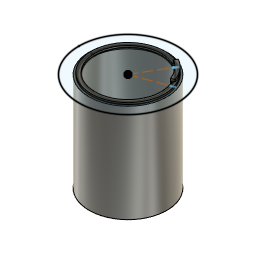
ex-vent v5 (Autodesk Fusion 360 design; units mm, degrees)
Autodesk Fusion 360 part; units mm, degrees
note: some values were not read from the file. Chosen so that the rebuilt part matches the saved one: the hand of a thread or coil.
sketch "Sketch1" plane through (0, 0, 0) normal (0, 0, 1) x (1, 0, 0)
  circle A0 centre (0, 0) radius 75.5
  circle A1 centre (0, 0) radius 79
  circle A2 centre (0, 0) radius 70
  line L0 (-75.5, 0) -> (75.5, 0)
  circle A3 centre (0, 0) radius 100
  dimension "ductid" = 151
  dimension "ductod" = 158
  dimension "d3" = 140
  dimension "d43" = 200
  constraint coincident A0.centre A1.centre
  constraint concentric A0 A2
  constraint coincident A0 L0.start
  constraint coincident A0 L0.end
  constraint horizontal L0
  constraint concentric A2 A3
  measures "ductid" diameter of A0
  measures "ductod" diameter of A1
  measures "d3" diameter of A2
  measures "d43" diameter of A3
extrude "Extrude1" add sketch "Sketch1" along normal blind 200 contours A1
sketch "Sketch2" plane through (0, 0, 200) normal (0, 0, 1) x (-1, 0, 0)
  circle A0 centre (0, 0) radius 75.5
  circle A1 centre (0, 0) radius 79
  circle A2 centre (0, 0) radius 75
  circle A3 centre (0, 0) radius 100
  circle A4 centre (0, 0) radius 72.5
  circle A5 centre (0, 0) radius 67.5
  circle A6 centre (0, 0) radius 69 construction
  arc A7 (-64.8289, -23.6266) -> (-34.4749, -59.7702) centre (0, 0) ccw
  line L0 (0, 0) -> (-64.8289, -23.6266) construction
  line L1 (0, 0) -> (-34.4749, -59.7702) construction
  line L2 (-64.8289, -23.6266) -> (-63.4196, -23.113)
  line L3 (-34.4749, -59.7702) -> (-33.7255, -58.4709)
  line L4 (-33.7255, -58.4709) -> (-36.2236, -62.8021)
  line L5 (-35.0164, -57.707) -> (-37.5152, -62.0392)
  line L6 (-36.2658, -59.8731) -> (-34.9745, -60.6365) construction
  line L7 (-63.4196, -23.113) -> (-68.1173, -24.8251)
  line L8 (-33.7255, -58.4709) -> (-37.5424, -64.9274)
  line L9 (-35.0164, -57.707) -> (-38.7645, -64.2052)
  line L10 (-63.4196, -23.113) -> (-70.4662, -25.6811)
  dimension "d13" = 200
  dimension "d14" = 145
  dimension "d17" = 150
  dimension "d20" = 135
  dimension "d21" = 138
  dimension "d22" = 40
  dimension "d23" = 1.5
  constraint coincident A0.centre A1.centre
  constraint concentric A2 A3
  constraint concentric A3 A5
  constraint coincident A6 A7.start
  constraint coincident A5 L2.end
  constraint coincident L0 L2.end
  constraint coincident L1 L3.end
  constraint coincident A5 L3.end
  constraint coincident A4 L4.end
  constraint parallel L3 L4
  constraint coincident A5 L5.start
  constraint coincident A4 L5.end
  constraint parallel L4 L5
  constraint midpoint L5 L6.start
  constraint midpoint L4 L6.end
  constraint coincident A4 L7.end
  constraint parallel L2 L7
  constraint coincident A2 L8.end
  constraint perpendicular L6 L8
  constraint coincident A2 L9.end
  constraint parallel L5 L9
  constraint coincident A2 L10.end
  constraint parallel L7 L10
  measures "d13" diameter of A3
  measures "d14" diameter of A4
  measures "d17" diameter of A2
  measures "d20" diameter of A5
  measures "d21" diameter of A6
  measures "d22" angle of L0 L1
  measures "d23" distance of L6.start L6.end
extrude "Extrude2" add sketch "Sketch2" against normal blind 5 contours A0 | A2 A4 L8 L10 | A2 A4 L9 L10 | A2 A4 L8 L9
extrude "Extrude3" add sketch "Sketch2" along normal blind 3.5 contours A2 A4 L8 L10 | A2 A4 L9 L10 | A2 A4 L8 L9 | A4 A7 L5 L7 L9 L10 | A4 A5 L2 L3 L4 L7 L10 | A4 A7 L4 L8 | A4 A7 L5 L8 L9 | A5 A7 L2 L5 L7 L9 L10 | A7 L3 L4 L8 | A5 A7 L5 L8 L9
extrude "Extrude4" add sketch "Sketch2" along normal blind 5.8 from surface at 3.5 contours A2 A4 L8 L9 | A4 A7 L5 L8 L9 | A5 A7 L2 L5 L7 L9 L10 | A5 A7 L5 L8 L9
extrude "Extrude5" add sketch "Sketch2" along normal blind 4.2 from surface at 9.3 contours A2 A4 L9 L10 | A2 A4 L8 L9 | A4 A7 L5 L7 L9 L10 | A4 A7 L5 L8 L9 | A5 A7 L2 L5 L7 L9 L10 | A5 A7 L5 L8 L9
chamfer "Chamfer3" distance 3 angle 45 1 edges at (-70.3907, -27.302, 195)
chamfer "Chamfer4" distance 5 angle 45 1 edges at (67.5937, -26.2171, 200)
coil "CoilPrimitive1" add diameter 150 section triangle in size 6 on centre turns 4 pitch 5 left hand placed x (1, 0, 0) y (0, 1, 0) z (0, 0, 1) at (0, 0, 0)
extrude "Extrude6" cut sketch "Sketch1" against normal blind 5 contours A0 A2 L0 | A0 A2 L0 | A2 L0 | A2 L0 | A1 | A3
fillet "Fillet3" radius 1.75 1 edges at (73.75, 0, 1.0104)
thread "Thread1" [rolled back] thread offset 0 thread length 25
fillet "Fillet1" [rolled back] radius 0.5
